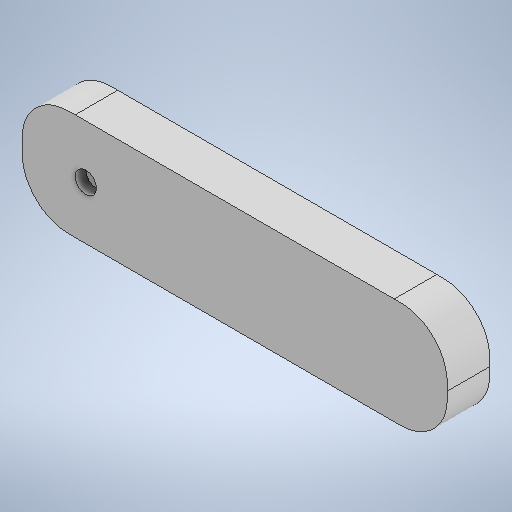
# Autodesk Inventor part: EjectorArm
Saved by Autodesk Inventor 2025.1 (Build 291241000, 241)
## iProperties
Created: 2025-02-22
Part Number: EjectorArm
Material: Generic
Document SubType Name: Modeling
Designer: 13156
Density: 1 g/cm^3
Appearance: Default
Author: 13156
Autodesk Inventor part; units mm, degrees
ref_plane "YZ Plane" through (0, 0, 0) normal (1, 0, 0) x (0, 1, 0)
ref_plane "XZ Plane" through (0, 0, 0) normal (0, 1, 0) x (-1, 0, 0)
ref_plane "XY Plane" through (0, 0, 0) normal (0, 0, 1) x (1, 0, 0)
sketch "Sketch5" plane through (0, 0, 0) normal (0, 0, 1) x (1, 0, 0)
  circle A0 centre (0, 0) radius 3.6
  line L0 (0, 0) -> (15.95, 0) construction
  circle A1 centre (15.95, 0) radius 2.4
  line L1 (0.2708, 3.5898) -> (16.1306, 2.3932)
  line L2 (0.2708, -3.5898) -> (16.1306, -2.3932)
  line L3 (5.6, 3.1877) -> (5.6, -3.1877)
  line L4 (0, 0) -> (-3.6, 0) construction
  circle A2 centre (0, 0) radius 1.55
  circle A3 centre (15.95, 0) radius 0.85
  circle A4 centre (0, 0) radius 2.975
  line L5 (-6, -5) -> (34, -5)
  line L6 (34, -5) -> (34, 5)
  line L7 (34, 5) -> (-6, 5)
  line L8 (-6, 5) -> (-6, -5)
  line L9 (0, 0) -> (0, -15.6524) construction
  line L10 (0, 0) -> (28.8257, 0) construction
  circle A5 centre (0, 0) radius 1
  dimension "d28" = 7.2
  dimension "d29" = 4.8
  dimension "d30" = 15.95
  dimension "d31" = 9.2
  dimension "d32" = 3.1
  dimension "d33" = 1.7
  dimension "d34" = 5.95
  dimension "d35" = 0
  dimension "d36" = 6
  dimension "d37" = 5
  dimension "d38" = 40
  dimension "d39" = 5
  dimension "d40" = 2
  constraints: 23 end point, 6 centre point, 5 coincident, 5 point on circle, 4 horizontal, 4 tangent, 2 parallel, 2 perpendicular, 2 point on line, 1 vertical, 1 other
  measures "d28" diameter of A0
  measures "d29" diameter of A1
  measures "d30" distance of L0.end point (0, 0)
  measures "d31" distance from line of L4.end L3
  measures "d32" diameter of A2
  measures "d33" diameter of A3
  measures "d34" diameter of A4
  measures "d35" distance of L9.start point (0, 0)
  measures "d36" distance from line of point (0, 0) L8
  measures "d37" distance from line of point (0, 0) L5
  measures "d38" distance of L5.start L5.end
  measures "d39" distance from line of point (0, 0) L7
  measures "d40" diameter of A5
extrude "Extrusion5" add sketch "Sketch5" along normal blind 4 contours A0 | A0 L1 L3 L2 | L1 A1 L2 L3 | A1 | A2 | A3 | A4 | L8 L7 L6 L5
extrude "Extrusion6" cut sketch "Sketch5" along normal blind 2 contours A0 | A0 L1 L3 L2 | L1 A1 L2 L3 | A1 | A2 | A3 | A4 | A5
extrude "Extrusion7" cut sketch "Sketch5" along normal blind 3 contours A0 | A0 L1 L3 L2 | A2 | A4 | A5
chamfer "Chamfer1" distance 1 angle 45 1 edges at (5.6, 0, 2)
fillet "Fillet2" radius 5 4 edges at (34, 5, 2) (34, -5, 2) (-6, -5, 2) (-6, 5, 2) curvature continuous yes
body "Solid3"
